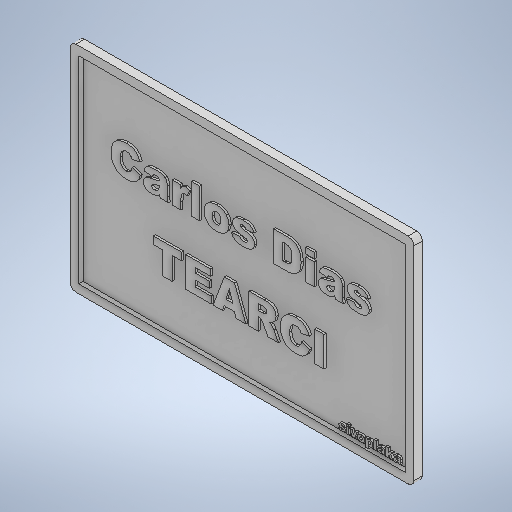
# Autodesk Inventor part: ID
Saved by Autodesk Inventor 2025.2 (Build 292293000, 293)
## iProperties
Created: 2025-01-22
Part Number: ID
Material: Generic
Document SubType Name: Modeling
Designer: Tony Dias
Density: 1 g/cm^3
Appearance: Default
Author: Tony Dias
## iProperties of the stored document ID_3DPrint.ipt
Created: 2025-01-22
Part Number: ID_3DPrint
Material: Generic
Document SubType Name: Modeling
Designer: Tony Dias
Density: 1 g/cm^3
Appearance: Default
Author: Tony Dias
Autodesk Inventor part; units mm, degrees
ref_plane "YZ Plane" through (0, 0, 0) normal (1, 0, 0) x (0, 1, 0)
ref_plane "XZ Plane" through (0, 0, 0) normal (0, 1, 0) x (-1, 0, 0)
ref_plane "XY Plane" through (0, 0, 0) normal (0, 0, 1) x (1, 0, 0)
sketch "Sketch1" plane through (0, 0, 0) normal (0, 0, 1) x (1, 0, 0)
  line L0 (-4, 2.5) -> (4, 2.5)
  line L1 (4, 2.5) -> (4, -2.5)
  line L2 (4, -2.5) -> (-4, -2.5)
  line L3 (-4, -2.5) -> (-4, 2.5)
  line L4 (-4, 2.5) -> (4, -2.5) construction
  line L5 (4, 2.5) -> (-4, -2.5) construction
  line L6 (-3.75, 2.3438) -> (3.75, -2.3438) construction
  line L7 (3.75, 2.3438) -> (-3.75, -2.3438) construction
  line L8 (3.8, -2.3) -> (-3.8, -2.3)
  line L9 (-3.8, 2.3) -> (-3.8, -2.3)
  line L10 (-3.8, 2.3) -> (3.8, 2.3)
  line L11 (3.8, 2.3) -> (3.8, -2.3)
  point P0 (0, 0)
  dimension "d0" = 8
  dimension "d1" = 5
  dimension "d2" = 7.5
  constraints: 24 end point, 4 midpoint, 3 horizontal, 3 perpendicular, 2 parallel, 1 point on line
  measures "d0" distance of L1.end L2.end
  measures "d1" distance of L0.end L1.end
  measures "d2" distance of L6.end L7.end
extrude "Extrusion1" add sketch "Sketch1" along normal blind 0.1 contours L8 L9 L10 L11
extrude "Extrusion2" add sketch "Sketch1" along normal blind 0.2
sketch "Sketch2" plane through (0, 0, 0) normal (0, 0, -1) x (-1, 0, 0)
  line L0 (-4, -2.5) -> (-4, 2.5) projected
  line L1 (-0.95, 0.4603) -> (-0.95, -0.4603) construction
  line L2 (-1.2, 0.4603) -> (-1.2, -0.4603)
  line L3 (-0.7, -0.4603) -> (-0.7, 0.4603)
  arc A0 (-0.7, 0.4603) -> (-1.2, 0.4603) centre (-0.95, 0.4603) ccw
  arc A1 (-1.2, -0.4603) -> (-0.7, -0.4603) centre (-0.95, -0.4603) ccw
  line L4 (0.95, 0.4603) -> (0.95, -0.4603) construction
  line L5 (0.7, 0.4603) -> (0.7, -0.4603)
  line L6 (1.2, -0.4603) -> (1.2, 0.4603)
  arc A2 (1.2, 0.4603) -> (0.7, 0.4603) centre (0.95, 0.4603) ccw
  arc A3 (0.7, -0.4603) -> (1.2, -0.4603) centre (0.95, -0.4603) ccw
  point P0 (0, 0)
  dimension "d13" = 0.5
  dimension "d15" = 0.5
  constraints: 16 end point, 8 point on circle, 8 tangent, 4 centre point, 2 parallel, 1 vertical
  measures "d13" diameter of A1
  measures "d15" diameter of A3
extrude "Extrusion3" add sketch "Sketch2" along normal blind 0.5
sketch "Sketch3" plane through (-1.2, -0.4603, 0) normal (-1, 0, 0) x (0, 0, 1)
  point P0 (0, 0.4603)
  point P1 (-0.2541, 0.4313)
hole "Hole1" at (-1.2, -0.029, -0.2541) direction (1, 0, 0) diameter 0.2 end through all
fillet "Face Fillet1" radius 0.133 1 edges at (0.95, 0.7103, -0.5)
fillet "Face Fillet2" radius 0.133 1 edges at (-0.95, 0.7103, -0.5)
sketch "Sketch4" plane through (0, 0, 0.2) normal (0, 0, 1) x (1, 0, 0)
  line L0 (-3.8117, 2.3101) -> (3.8117, 2.3101) construction
  line L1 (3.8117, 2.3101) -> (3.8117, -2.2966) construction
  line L2 (3.8117, -2.2966) -> (-3.8117, -2.2966) construction
  line L3 (-3.8117, -2.2966) -> (-3.8117, 2.3101) construction
  line L4 (2.2708, -1.8777) -> (3.7723, -1.8777) construction
  line L5 (3.7723, -1.8777) -> (3.7723, -2.2813) construction
  line L6 (3.7723, -2.2813) -> (2.2708, -2.2813) construction
  line L7 (2.2708, -2.2813) -> (2.2708, -1.8777) construction
  line L8 (-2.5069, 0.7143) -> (-2.3176, 0.657)
  spline S0 degree 2 poles (-2.3176, 0.657) (-2.3365, 0.5775) (-2.4187, 0.4704) (-2.5406, 0.4159) (-2.6343, 0.4159) knots 0 0 0 1 2 3 3 3
  spline S1 degree 2 poles (-2.6343, 0.4159) (-2.7488, 0.4159) (-2.893, 0.4826) (-2.9981, 0.6496) (-2.9981, 0.7797) knots 0 0 0 1 2 3 3 3
  spline S2 degree 2 poles (-2.9981, 0.7797) (-2.9981, 0.9535) (-2.8135, 1.1401) (-2.6444, 1.1401) knots 0 0 0 1 2 2 2
  spline S3 degree 2 poles (-2.6444, 1.1401) (-2.5123, 1.1401) (-2.3614, 1.033) (-2.3244, 0.9225) knots 0 0 0 1 2 2 2
  line L9 (-2.3244, 0.9225) -> (-2.5157, 0.8801)
  spline S4 degree 2 poles (-2.5157, 0.8801) (-2.5258, 0.9117) (-2.5366, 0.9265) knots 0 0 0 1 1 1
  spline S5 degree 2 poles (-2.5366, 0.9265) (-2.5548, 0.9515) (-2.6073, 0.9784) (-2.6397, 0.9784) knots 0 0 0 1 2 2 2
  spline S6 degree 2 poles (-2.6397, 0.9784) (-2.7124, 0.9784) (-2.7515, 0.9191) knots 0 0 0 1 1 1
  spline S7 degree 2 poles (-2.7515, 0.9191) (-2.7811, 0.8753) (-2.7811, 0.781) knots 0 0 0 1 1 1
  spline S8 degree 2 poles (-2.7811, 0.781) (-2.7811, 0.6645) (-2.7104, 0.5782) (-2.6464, 0.5782) knots 0 0 0 1 2 2 2
  spline S9 degree 2 poles (-2.6464, 0.5782) (-2.5844, 0.5782) (-2.5211, 0.6476) (-2.5069, 0.7143) knots 0 0 0 1 2 2 2
  line L10 (-2.0468, 0.7702) -> (-2.2327, 0.7898)
  spline S10 degree 2 poles (-2.2327, 0.7898) (-2.2219, 0.839) (-2.1829, 0.8949) (-2.1451, 0.9158) knots 0 0 0 1 2 2 2
  spline S11 degree 2 poles (-2.1451, 0.9158) (-2.1189, 0.9306) (-2.0252, 0.9468) (-1.9706, 0.9468) knots 0 0 0 1 2 2 2
  spline S12 degree 2 poles (-1.9706, 0.9468) (-1.8837, 0.9468) (-1.778, 0.9272) (-1.7423, 0.8962) knots 0 0 0 1 2 2 2
  spline S13 degree 2 poles (-1.7423, 0.8962) (-1.7173, 0.8747) (-1.689, 0.7958) (-1.689, 0.7601) knots 0 0 0 1 2 2 2
  line L11 (-1.689, 0.7601) -> (-1.689, 0.5358)
  spline S14 degree 2 poles (-1.689, 0.5358) (-1.689, 0.5001) (-1.6803, 0.4596) (-1.6648, 0.428) knots 0 0 0 1 2 2 2
  line L12 (-1.6648, 0.428) -> (-1.8474, 0.428)
  spline S15 degree 2 poles (-1.8474, 0.428) (-1.8581, 0.4475) (-1.8649, 0.4677) (-1.8682, 0.49) knots 0 0 0 1 2 2 2
  spline S16 degree 2 poles (-1.8682, 0.49) (-1.906, 0.4536) (-1.9437, 0.4374) knots 0 0 0 1 1 1
  spline S17 degree 2 poles (-1.9437, 0.4374) (-1.9956, 0.4165) (-2.0636, 0.4165) knots 0 0 0 1 1 1
  spline S18 degree 2 poles (-2.0636, 0.4165) (-2.1546, 0.4165) (-2.2482, 0.5007) (-2.2482, 0.5621) knots 0 0 0 1 2 2 2
  spline S19 degree 2 poles (-2.2482, 0.5621) (-2.2482, 0.62) (-2.2145, 0.657) knots 0 0 0 1 1 1
  spline S20 degree 2 poles (-2.2145, 0.657) (-2.1802, 0.6941) (-2.0892, 0.7123) knots 0 0 0 1 1 1
  spline S21 degree 2 poles (-2.0892, 0.7123) (-1.9801, 0.7345) (-1.9154, 0.752) (-1.879, 0.7662) knots 0 0 0 1 2 2 2
  spline S22 degree 2 poles (-1.879, 0.7662) (-1.879, 0.8019) (-1.9087, 0.8309) (-1.9457, 0.8309) knots 0 0 0 1 2 2 2
  spline S23 degree 2 poles (-1.9457, 0.8309) (-1.9929, 0.8309) (-2.0171, 0.8154) knots 0 0 0 1 1 1
  spline S24 degree 2 poles (-2.0171, 0.8154) (-2.0353, 0.8032) (-2.0468, 0.7702) knots 0 0 0 1 1 1
  spline S25 degree 2 poles (-1.879, 0.6685) (-1.9188, 0.6544) (-1.9626, 0.6429) knots 0 0 0 1 1 1
  spline S26 degree 2 poles (-1.9626, 0.6429) (-2.0218, 0.6274) (-2.0373, 0.6119) knots 0 0 0 1 1 1
  spline S27 degree 2 poles (-2.0373, 0.6119) (-2.0535, 0.5964) (-2.0535, 0.5762) knots 0 0 0 1 1 1
  spline S28 degree 2 poles (-2.0535, 0.5762) (-2.0535, 0.5533) (-2.0218, 0.5243) (-1.9909, 0.5243) knots 0 0 0 1 2 2 2
  spline S29 degree 2 poles (-1.9909, 0.5243) (-1.9578, 0.5243) (-1.9026, 0.556) (-1.879, 0.6011) (-1.879, 0.6375) knots 0 0 0 1 2 3 3 3
  line L13 (-1.879, 0.6375) -> (-1.879, 0.6685)
  line L14 (-1.5698, 0.9353) -> (-1.3879, 0.9353)
  line L15 (-1.3879, 0.9353) -> (-1.3879, 0.8524)
  spline S30 degree 2 poles (-1.3879, 0.8524) (-1.3616, 0.9063) (-1.3057, 0.9468) (-1.2646, 0.9468) knots 0 0 0 1 2 2 2
  spline S31 degree 2 poles (-1.2646, 0.9468) (-1.2215, 0.9468) (-1.1703, 0.9198) knots 0 0 0 1 1 1
  line L16 (-1.1703, 0.9198) -> (-1.2302, 0.7817)
  spline S32 degree 2 poles (-1.2302, 0.7817) (-1.2646, 0.7958) (-1.2848, 0.7958) knots 0 0 0 1 1 1
  spline S33 degree 2 poles (-1.2848, 0.7958) (-1.3232, 0.7958) (-1.3441, 0.7642) knots 0 0 0 1 1 1
  spline S34 degree 2 poles (-1.3441, 0.7642) (-1.3744, 0.7197) (-1.3744, 0.5978) knots 0 0 0 1 1 1
  line L17 (-1.3744, 0.5978) -> (-1.3744, 0.428)
  line L18 (-1.3744, 0.428) -> (-1.5698, 0.428)
  line L19 (-1.5698, 0.428) -> (-1.5698, 0.9353)
  line L20 (-1.1305, 1.128) -> (-0.9358, 1.128)
  line L21 (-0.9358, 1.128) -> (-0.9358, 0.428)
  line L22 (-0.9358, 0.428) -> (-1.1305, 0.428)
  line L23 (-1.1305, 0.428) -> (-1.1305, 1.128)
  spline S35 degree 2 poles (-0.8347, 0.68) (-0.8347, 0.7965) (-0.6784, 0.9468) (-0.545, 0.9468) knots 0 0 0 1 2 2 2
  spline S36 degree 2 poles (-0.545, 0.9468) (-0.3928, 0.9468) (-0.3153, 0.8585) knots 0 0 0 1 1 1
  spline S37 degree 2 poles (-0.3153, 0.8585) (-0.2526, 0.7871) (-0.2526, 0.6833) knots 0 0 0 1 1 1
  spline S38 degree 2 poles (-0.2526, 0.6833) (-0.2526, 0.5661) (-0.4076, 0.4165) (-0.5444, 0.4165) knots 0 0 0 1 2 2 2
  spline S39 degree 2 poles (-0.5444, 0.4165) (-0.667, 0.4165) (-0.7424, 0.4785) knots 0 0 0 1 1 1
  spline S40 degree 2 poles (-0.7424, 0.4785) (-0.8347, 0.5553) (-0.8347, 0.68) knots 0 0 0 1 1 1
  spline S41 degree 2 poles (-0.64, 0.6806) (-0.64, 0.6126) (-0.5855, 0.5479) (-0.5437, 0.5479) knots 0 0 0 1 2 2 2
  spline S42 degree 2 poles (-0.5437, 0.5479) (-0.5019, 0.5479) (-0.448, 0.6119) (-0.448, 0.6827) knots 0 0 0 1 2 2 2
  spline S43 degree 2 poles (-0.448, 0.6827) (-0.448, 0.748) (-0.5026, 0.8127) (-0.5423, 0.8127) knots 0 0 0 1 2 2 2
  spline S44 degree 2 poles (-0.5423, 0.8127) (-0.5848, 0.8127) (-0.64, 0.7473) (-0.64, 0.6806) knots 0 0 0 1 2 2 2
  line L24 (-0.1927, 0.5688) -> (0, 0.587)
  spline S45 degree 2 poles (0, 0.587) (0.0121, 0.5526) (0.0552, 0.523) (0.091, 0.523) knots 0 0 0 1 2 2 2
  spline S46 degree 2 poles (0.091, 0.523) (0.1307, 0.523) (0.1523, 0.5398) knots 0 0 0 1 1 1
  spline S47 degree 2 poles (0.1523, 0.5398) (0.1691, 0.5519) (0.1691, 0.5708) knots 0 0 0 1 1 1
  spline S48 degree 2 poles (0.1691, 0.5708) (0.1691, 0.5917) (0.1469, 0.6032) knots 0 0 0 1 1 1
  spline S49 degree 2 poles (0.1469, 0.6032) (0.1307, 0.6112) (0.0633, 0.6234) knots 0 0 0 1 1 1
  spline S50 degree 2 poles (0.0633, 0.6234) (-0.0384, 0.6409) (-0.1172, 0.6712) (-0.1711, 0.7426) (-0.1711, 0.7884) knots 0 0 0 1 2 3 3 3
  spline S51 degree 2 poles (-0.1711, 0.7884) (-0.1711, 0.8383) (-0.1125, 0.911) (-0.0108, 0.9468) (0.0755, 0.9468) knots 0 0 0 1 2 3 3 3
  spline S52 degree 2 poles (0.0755, 0.9468) (0.1664, 0.9468) (0.2526, 0.9191) (0.3106, 0.8612) (0.3295, 0.8113) knots 0 0 0 1 2 3 3 3
  line L25 (0.3295, 0.8113) -> (0.1449, 0.7931)
  spline S53 degree 2 poles (0.1449, 0.7931) (0.1374, 0.8174) (0.1213, 0.8288) knots 0 0 0 1 1 1
  spline S54 degree 2 poles (0.1213, 0.8288) (0.0984, 0.8443) (0.0654, 0.8443) knots 0 0 0 1 1 1
  spline S55 degree 2 poles (0.0654, 0.8443) (0.033, 0.8443) (0.0027, 0.8208) (0.0027, 0.8039) knots 0 0 0 1 2 2 2
  spline S56 degree 2 poles (0.0027, 0.8039) (0.0027, 0.7857) (0.0222, 0.7763) knots 0 0 0 1 1 1
  spline S57 degree 2 poles (0.0222, 0.7763) (0.0411, 0.7662) (0.1051, 0.7588) knots 0 0 0 1 1 1
  spline S58 degree 2 poles (0.1051, 0.7588) (0.2021, 0.748) (0.2971, 0.7089) (0.347, 0.6362) (0.347, 0.593) knots 0 0 0 1 2 3 3 3
  spline S59 degree 2 poles (0.347, 0.593) (0.347, 0.5486) (0.2937, 0.4657) (0.1799, 0.4165) (0.0815, 0.4165) knots 0 0 0 1 2 3 3 3
  spline S60 degree 2 poles (0.0815, 0.4165) (-0.0579, 0.4165) (-0.1758, 0.496) (-0.1927, 0.5688) knots 0 0 0 1 2 2 2
  line L26 (0.7815, 1.128) -> (1.1029, 1.128)
  spline S61 degree 2 poles (1.1029, 1.128) (1.1979, 1.128) (1.3151, 1.0761) (1.3912, 0.9798) (1.4256, 0.8518) (1.4256, 0.7803) knots 0 0 0 1 2 3 4 4 4
  spline S62 degree 2 poles (1.4256, 0.7803) (1.4256, 0.6678) (1.3744, 0.5445) (1.2841, 0.461) (1.2316, 0.4468) knots 0 0 0 1 2 3 3 3
  spline S63 degree 2 poles (1.2316, 0.4468) (1.1608, 0.428) (1.1029, 0.428) knots 0 0 0 1 1 1
  line L27 (1.1029, 0.428) -> (0.7815, 0.428)
  line L28 (0.7815, 0.428) -> (0.7815, 1.128)
  line L29 (0.9978, 0.9697) -> (0.9978, 0.587)
  line L30 (0.9978, 0.587) -> (1.051, 0.587)
  spline S64 degree 2 poles (1.051, 0.587) (1.1184, 0.587) (1.1756, 0.6173) (1.208, 0.6921) (1.208, 0.7763) knots 0 0 0 1 2 3 3 3
  spline S65 degree 2 poles (1.208, 0.7763) (1.208, 0.8875) (1.1352, 0.9697) (1.0517, 0.9697) knots 0 0 0 1 2 2 2
  line L31 (1.0517, 0.9697) -> (0.9978, 0.9697)
  line L32 (1.5341, 0.9353) -> (1.7288, 0.9353)
  line L33 (1.7288, 0.9353) -> (1.7288, 0.428)
  line L34 (1.7288, 0.428) -> (1.5341, 0.428)
  line L35 (1.5341, 0.428) -> (1.5341, 0.9353)
  line L36 (1.5341, 1.128) -> (1.7288, 1.128)
  line L37 (1.7288, 1.128) -> (1.7288, 0.9959)
  line L38 (1.7288, 0.9959) -> (1.5341, 0.9959)
  line L39 (1.5341, 0.9959) -> (1.5341, 1.128)
  line L40 (2.0306, 0.7702) -> (1.8447, 0.7898)
  spline S66 degree 2 poles (1.8447, 0.7898) (1.8554, 0.839) (1.8945, 0.8949) (1.9322, 0.9158) knots 0 0 0 1 2 2 2
  spline S67 degree 2 poles (1.9322, 0.9158) (1.9585, 0.9306) (2.0522, 0.9468) (2.1067, 0.9468) knots 0 0 0 1 2 2 2
  spline S68 degree 2 poles (2.1067, 0.9468) (2.1936, 0.9468) (2.2994, 0.9272) (2.3351, 0.8962) knots 0 0 0 1 2 2 2
  spline S69 degree 2 poles (2.3351, 0.8962) (2.3601, 0.8747) (2.3884, 0.7958) (2.3884, 0.7601) knots 0 0 0 1 2 2 2
  line L41 (2.3884, 0.7601) -> (2.3884, 0.5358)
  spline S70 degree 2 poles (2.3884, 0.5358) (2.3884, 0.5001) (2.3971, 0.4596) (2.4126, 0.428) knots 0 0 0 1 2 2 2
  line L42 (2.4126, 0.428) -> (2.23, 0.428)
  spline S71 degree 2 poles (2.23, 0.428) (2.2192, 0.4475) (2.2125, 0.4677) (2.2091, 0.49) knots 0 0 0 1 2 2 2
  spline S72 degree 2 poles (2.2091, 0.49) (2.1714, 0.4536) (2.1337, 0.4374) knots 0 0 0 1 1 1
  spline S73 degree 2 poles (2.1337, 0.4374) (2.0818, 0.4165) (2.0138, 0.4165) knots 0 0 0 1 1 1
  spline S74 degree 2 poles (2.0138, 0.4165) (1.9228, 0.4165) (1.8292, 0.5007) (1.8292, 0.5621) knots 0 0 0 1 2 2 2
  spline S75 degree 2 poles (1.8292, 0.5621) (1.8292, 0.62) (1.8628, 0.657) knots 0 0 0 1 1 1
  spline S76 degree 2 poles (1.8628, 0.657) (1.8972, 0.6941) (1.9882, 0.7123) knots 0 0 0 1 1 1
  spline S77 degree 2 poles (1.9882, 0.7123) (2.0973, 0.7345) (2.162, 0.752) (2.1984, 0.7662) knots 0 0 0 1 2 2 2
  spline S78 degree 2 poles (2.1984, 0.7662) (2.1984, 0.8019) (2.1687, 0.8309) (2.1317, 0.8309) knots 0 0 0 1 2 2 2
  spline S79 degree 2 poles (2.1317, 0.8309) (2.0845, 0.8309) (2.0603, 0.8154) knots 0 0 0 1 1 1
  spline S80 degree 2 poles (2.0603, 0.8154) (2.0421, 0.8032) (2.0306, 0.7702) knots 0 0 0 1 1 1
  spline S81 degree 2 poles (2.1984, 0.6685) (2.1586, 0.6544) (2.1148, 0.6429) knots 0 0 0 1 1 1
  spline S82 degree 2 poles (2.1148, 0.6429) (2.0555, 0.6274) (2.04, 0.6119) knots 0 0 0 1 1 1
  spline S83 degree 2 poles (2.04, 0.6119) (2.0239, 0.5964) (2.0239, 0.5762) knots 0 0 0 1 1 1
  spline S84 degree 2 poles (2.0239, 0.5762) (2.0239, 0.5533) (2.0555, 0.5243) (2.0865, 0.5243) knots 0 0 0 1 2 2 2
  spline S85 degree 2 poles (2.0865, 0.5243) (2.1195, 0.5243) (2.1748, 0.556) (2.1984, 0.6011) (2.1984, 0.6375) knots 0 0 0 1 2 3 3 3
  line L43 (2.1984, 0.6375) -> (2.1984, 0.6685)
  line L44 (2.4712, 0.5688) -> (2.6639, 0.587)
  spline S86 degree 2 poles (2.6639, 0.587) (2.676, 0.5526) (2.7192, 0.523) (2.7549, 0.523) knots 0 0 0 1 2 2 2
  spline S87 degree 2 poles (2.7549, 0.523) (2.7946, 0.523) (2.8162, 0.5398) knots 0 0 0 1 1 1
  spline S88 degree 2 poles (2.8162, 0.5398) (2.833, 0.5519) (2.833, 0.5708) knots 0 0 0 1 1 1
  spline S89 degree 2 poles (2.833, 0.5708) (2.833, 0.5917) (2.8108, 0.6032) knots 0 0 0 1 1 1
  spline S90 degree 2 poles (2.8108, 0.6032) (2.7946, 0.6112) (2.7272, 0.6234) knots 0 0 0 1 1 1
  spline S91 degree 2 poles (2.7272, 0.6234) (2.6255, 0.6409) (2.5467, 0.6712) (2.4928, 0.7426) (2.4928, 0.7884) knots 0 0 0 1 2 3 3 3
  spline S92 degree 2 poles (2.4928, 0.7884) (2.4928, 0.8383) (2.5514, 0.911) (2.6531, 0.9468) (2.7394, 0.9468) knots 0 0 0 1 2 3 3 3
  spline S93 degree 2 poles (2.7394, 0.9468) (2.8303, 0.9468) (2.9166, 0.9191) (2.9745, 0.8612) (2.9934, 0.8113) knots 0 0 0 1 2 3 3 3
  line L45 (2.9934, 0.8113) -> (2.8088, 0.7931)
  spline S94 degree 2 poles (2.8088, 0.7931) (2.8013, 0.8174) (2.7852, 0.8288) knots 0 0 0 1 1 1
  spline S95 degree 2 poles (2.7852, 0.8288) (2.7623, 0.8443) (2.7293, 0.8443) knots 0 0 0 1 1 1
  spline S96 degree 2 poles (2.7293, 0.8443) (2.6969, 0.8443) (2.6666, 0.8208) (2.6666, 0.8039) knots 0 0 0 1 2 2 2
  spline S97 degree 2 poles (2.6666, 0.8039) (2.6666, 0.7857) (2.6861, 0.7763) knots 0 0 0 1 1 1
  spline S98 degree 2 poles (2.6861, 0.7763) (2.705, 0.7662) (2.769, 0.7588) knots 0 0 0 1 1 1
  spline S99 degree 2 poles (2.769, 0.7588) (2.866, 0.748) (2.961, 0.7089) (3.0109, 0.6362) (3.0109, 0.593) knots 0 0 0 1 2 3 3 3
  spline S100 degree 2 poles (3.0109, 0.593) (3.0109, 0.5486) (2.9577, 0.4657) (2.8438, 0.4165) (2.7454, 0.4165) knots 0 0 0 1 2 3 3 3
  spline S101 degree 2 poles (2.7454, 0.4165) (2.606, 0.4165) (2.4881, 0.496) (2.4712, 0.5688) knots 0 0 0 1 2 2 2
  line L46 (-2.0168, -0.4144) -> (-1.3586, -0.4144)
  line L47 (-1.3586, -0.4144) -> (-1.3586, -0.5875)
  line L48 (-1.3586, -0.5875) -> (-1.5795, -0.5875)
  line L49 (-1.5795, -0.5875) -> (-1.5795, -1.1144)
  line L50 (-1.5795, -1.1144) -> (-1.7958, -1.1144)
  line L51 (-1.7958, -1.1144) -> (-1.7958, -0.5875)
  line L52 (-1.7958, -0.5875) -> (-2.0168, -0.5875)
  line L53 (-2.0168, -0.5875) -> (-2.0168, -0.4144)
  line L54 (-1.2609, -0.4144) -> (-0.6815, -0.4144)
  line L55 (-0.6815, -0.4144) -> (-0.6815, -0.564)
  line L56 (-0.6815, -0.564) -> (-1.0439, -0.564)
  line L57 (-1.0439, -0.564) -> (-1.0439, -0.6751)
  line L58 (-1.0439, -0.6751) -> (-0.7077, -0.6751)
  line L59 (-0.7077, -0.6751) -> (-0.7077, -0.818)
  line L60 (-0.7077, -0.818) -> (-1.0439, -0.818)
  line L61 (-1.0439, -0.818) -> (-1.0439, -0.9561)
  line L62 (-1.0439, -0.9561) -> (-0.6707, -0.9561)
  line L63 (-0.6707, -0.9561) -> (-0.6707, -1.1144)
  line L64 (-0.6707, -1.1144) -> (-1.2609, -1.1144)
  line L65 (-1.2609, -1.1144) -> (-1.2609, -0.4144)
  line L66 (-0.1236, -0.9985) -> (-0.3695, -0.9985)
  line L67 (-0.3695, -0.9985) -> (-0.4039, -1.1144)
  line L68 (-0.4039, -1.1144) -> (-0.6249, -1.1144)
  line L69 (-0.6249, -1.1144) -> (-0.3615, -0.4144)
  line L70 (-0.3615, -0.4144) -> (-0.125, -0.4144)
  line L71 (-0.125, -0.4144) -> (0.1378, -1.1144)
  line L72 (0.1378, -1.1144) -> (-0.0886, -1.1144)
  line L73 (-0.0886, -1.1144) -> (-0.1236, -0.9985)
  line L74 (-0.1688, -0.8469) -> (-0.2456, -0.5956)
  line L75 (-0.2456, -0.5956) -> (-0.3224, -0.8469)
  line L76 (-0.3224, -0.8469) -> (-0.1688, -0.8469)
  line L77 (0.2105, -1.1144) -> (0.2105, -0.4144)
  line L78 (0.2105, -0.4144) -> (0.571, -0.4144)
  spline S102 degree 2 poles (0.571, -0.4144) (0.6707, -0.4144) (0.7771, -0.4488) (0.8418, -0.5417) (0.8418, -0.6084) knots 0 0 0 1 2 3 3 3
  spline S103 degree 2 poles (0.8418, -0.6084) (0.8418, -0.667) (0.792, -0.7513) (0.7488, -0.7775) knots 0 0 0 1 2 2 2
  spline S104 degree 2 poles (0.7488, -0.7775) (0.7212, -0.7944) (0.6727, -0.8052) knots 0 0 0 1 1 1
  spline S105 degree 2 poles (0.6727, -0.8052) (0.7111, -0.818) (0.7293, -0.8308) knots 0 0 0 1 1 1
  spline S106 degree 2 poles (0.7293, -0.8308) (0.7408, -0.8395) (0.7859, -0.8961) (0.794, -0.9116) knots 0 0 0 1 2 2 2
  line L79 (0.794, -0.9116) -> (0.8984, -1.1144)
  line L80 (0.8984, -1.1144) -> (0.6538, -1.1144)
  line L81 (0.6538, -1.1144) -> (0.5386, -0.9001)
  spline S107 degree 2 poles (0.5386, -0.9001) (0.5171, -0.8591) (0.5002, -0.8463) knots 0 0 0 1 1 1
  spline S108 degree 2 poles (0.5002, -0.8463) (0.4767, -0.8301) (0.447, -0.8301) knots 0 0 0 1 1 1
  line L82 (0.447, -0.8301) -> (0.4282, -0.8301)
  line L83 (0.4282, -0.8301) -> (0.4282, -1.1144)
  line L84 (0.4282, -1.1144) -> (0.2105, -1.1144)
  line L85 (0.4282, -0.698) -> (0.5191, -0.698)
  spline S109 degree 2 poles (0.5191, -0.698) (0.5333, -0.698) (0.5757, -0.6886) knots 0 0 0 1 1 1
  spline S110 degree 2 poles (0.5757, -0.6886) (0.5973, -0.6839) (0.6242, -0.6488) (0.6242, -0.6259) knots 0 0 0 1 2 2 2
  spline S111 degree 2 poles (0.6242, -0.6259) (0.6242, -0.5923) (0.5818, -0.5559) (0.5225, -0.5559) knots 0 0 0 1 2 2 2
  line L86 (0.5225, -0.5559) -> (0.4282, -0.5559)
  line L87 (0.4282, -0.5559) -> (0.4282, -0.698)
  line L88 (1.4347, -0.8281) -> (1.624, -0.8853)
  spline S112 degree 2 poles (1.624, -0.8853) (1.6051, -0.9648) (1.523, -1.0719) (1.401, -1.1265) (1.3074, -1.1265) knots 0 0 0 1 2 3 3 3
  spline S113 degree 2 poles (1.3074, -1.1265) (1.1928, -1.1265) (1.0487, -1.0598) (0.9436, -0.8927) (0.9436, -0.7627) knots 0 0 0 1 2 3 3 3
  spline S114 degree 2 poles (0.9436, -0.7627) (0.9436, -0.5889) (1.1282, -0.4023) (1.2973, -0.4023) knots 0 0 0 1 2 2 2
  spline S115 degree 2 poles (1.2973, -0.4023) (1.4293, -0.4023) (1.5802, -0.5094) (1.6173, -0.6199) knots 0 0 0 1 2 2 2
  line L89 (1.6173, -0.6199) -> (1.4259, -0.6623)
  spline S116 degree 2 poles (1.4259, -0.6623) (1.4158, -0.6307) (1.4051, -0.6158) knots 0 0 0 1 1 1
  spline S117 degree 2 poles (1.4051, -0.6158) (1.3869, -0.5909) (1.3343, -0.564) (1.302, -0.564) knots 0 0 0 1 2 2 2
  spline S118 degree 2 poles (1.302, -0.564) (1.2292, -0.564) (1.1901, -0.6232) knots 0 0 0 1 1 1
  spline S119 degree 2 poles (1.1901, -0.6232) (1.1605, -0.667) (1.1605, -0.7614) knots 0 0 0 1 1 1
  spline S120 degree 2 poles (1.1605, -0.7614) (1.1605, -0.8779) (1.2312, -0.9642) (1.2952, -0.9642) knots 0 0 0 1 2 2 2
  spline S121 degree 2 poles (1.2952, -0.9642) (1.3572, -0.9642) (1.4205, -0.8948) (1.4347, -0.8281) knots 0 0 0 1 2 2 2
  line L90 (1.7385, -0.4144) -> (1.9555, -0.4144)
  line L91 (1.9555, -0.4144) -> (1.9555, -1.1144)
  line L92 (1.9555, -1.1144) -> (1.7385, -1.1144)
  line L93 (1.7385, -1.1144) -> (1.7385, -0.4144)
  line L94 (2.2983, -2.1117) -> (2.3533, -2.1065)
  spline S122 degree 2 poles (2.3533, -2.1065) (2.3568, -2.1163) (2.3691, -2.1248) (2.3793, -2.1248) knots 0 0 0 1 2 2 2
  spline S123 degree 2 poles (2.3793, -2.1248) (2.3907, -2.1248) (2.3968, -2.12) knots 0 0 0 1 1 1
  spline S124 degree 2 poles (2.3968, -2.12) (2.4017, -2.1165) (2.4017, -2.1111) knots 0 0 0 1 1 1
  spline S125 degree 2 poles (2.4017, -2.1111) (2.4017, -2.1052) (2.3953, -2.1019) knots 0 0 0 1 1 1
  spline S126 degree 2 poles (2.3953, -2.1019) (2.3907, -2.0996) (2.3714, -2.0961) knots 0 0 0 1 1 1
  spline S127 degree 2 poles (2.3714, -2.0961) (2.3424, -2.0911) (2.3198, -2.0825) (2.3044, -2.0621) (2.3044, -2.049) knots 0 0 0 1 2 3 3 3
  spline S128 degree 2 poles (2.3044, -2.049) (2.3044, -2.0347) (2.3212, -2.0139) (2.3503, -2.0037) (2.3749, -2.0037) knots 0 0 0 1 2 3 3 3
  spline S129 degree 2 poles (2.3749, -2.0037) (2.4009, -2.0037) (2.4255, -2.0116) (2.4421, -2.0282) (2.4475, -2.0424) knots 0 0 0 1 2 3 3 3
  line L95 (2.4475, -2.0424) -> (2.3947, -2.0476)
  spline S130 degree 2 poles (2.3947, -2.0476) (2.3926, -2.0407) (2.388, -2.0374) knots 0 0 0 1 1 1
  spline S131 degree 2 poles (2.388, -2.0374) (2.3814, -2.033) (2.372, -2.033) knots 0 0 0 1 1 1
  spline S132 degree 2 poles (2.372, -2.033) (2.3628, -2.033) (2.3541, -2.0397) (2.3541, -2.0445) knots 0 0 0 1 2 2 2
  spline S133 degree 2 poles (2.3541, -2.0445) (2.3541, -2.0497) (2.3597, -2.0524) knots 0 0 0 1 1 1
  spline S134 degree 2 poles (2.3597, -2.0524) (2.3651, -2.0553) (2.3834, -2.0574) knots 0 0 0 1 1 1
  spline S135 degree 2 poles (2.3834, -2.0574) (2.4111, -2.0605) (2.4382, -2.0717) (2.4525, -2.0925) (2.4525, -2.1048) knots 0 0 0 1 2 3 3 3
  spline S136 degree 2 poles (2.4525, -2.1048) (2.4525, -2.1175) (2.4373, -2.1412) (2.4047, -2.1552) (2.3766, -2.1552) knots 0 0 0 1 2 3 3 3
  spline S137 degree 2 poles (2.3766, -2.1552) (2.3368, -2.1552) (2.3031, -2.1325) (2.2983, -2.1117) knots 0 0 0 1 2 2 2
  line L96 (2.481, -2.007) -> (2.5366, -2.007)
  line L97 (2.5366, -2.007) -> (2.5366, -2.152)
  line L98 (2.5366, -2.152) -> (2.481, -2.152)
  line L99 (2.481, -2.152) -> (2.481, -2.007)
  line L100 (2.481, -1.952) -> (2.5366, -1.952)
  line L101 (2.5366, -1.952) -> (2.5366, -1.9897)
  line L102 (2.5366, -1.9897) -> (2.481, -1.9897)
  line L103 (2.481, -1.9897) -> (2.481, -1.952)
  line L104 (2.5556, -2.007) -> (2.6134, -2.007)
  line L105 (2.6134, -2.007) -> (2.6417, -2.0988)
  line L106 (2.6417, -2.0988) -> (2.6708, -2.007)
  line L107 (2.6708, -2.007) -> (2.7268, -2.007)
  line L108 (2.7268, -2.007) -> (2.6652, -2.152)
  line L109 (2.6652, -2.152) -> (2.6159, -2.152)
  line L110 (2.6159, -2.152) -> (2.5556, -2.007)
  spline S138 degree 2 poles (2.736, -2.08) (2.736, -2.0467) (2.7807, -2.0037) (2.8188, -2.0037) knots 0 0 0 1 2 2 2
  spline S139 degree 2 poles (2.8188, -2.0037) (2.8623, -2.0037) (2.8844, -2.0289) knots 0 0 0 1 1 1
  spline S140 degree 2 poles (2.8844, -2.0289) (2.9023, -2.0494) (2.9023, -2.079) knots 0 0 0 1 1 1
  spline S141 degree 2 poles (2.9023, -2.079) (2.9023, -2.1125) (2.8581, -2.1552) (2.819, -2.1552) knots 0 0 0 1 2 2 2
  spline S142 degree 2 poles (2.819, -2.1552) (2.7839, -2.1552) (2.7624, -2.1375) knots 0 0 0 1 1 1
  spline S143 degree 2 poles (2.7624, -2.1375) (2.736, -2.1156) (2.736, -2.08) knots 0 0 0 1 1 1
  spline S144 degree 2 poles (2.7916, -2.0798) (2.7916, -2.0992) (2.8072, -2.1177) (2.8192, -2.1177) knots 0 0 0 1 2 2 2
  spline S145 degree 2 poles (2.8192, -2.1177) (2.8311, -2.1177) (2.8465, -2.0994) (2.8465, -2.0792) knots 0 0 0 1 2 2 2
  spline S146 degree 2 poles (2.8465, -2.0792) (2.8465, -2.0605) (2.8309, -2.042) (2.8196, -2.042) knots 0 0 0 1 2 2 2
  spline S147 degree 2 poles (2.8196, -2.042) (2.8074, -2.042) (2.7916, -2.0607) (2.7916, -2.0798) knots 0 0 0 1 2 2 2
  line L111 (2.9297, -2.207) -> (2.9297, -2.007)
  line L112 (2.9297, -2.007) -> (2.9816, -2.007)
  line L113 (2.9816, -2.007) -> (2.9816, -2.0284)
  spline S148 degree 2 poles (2.9816, -2.0284) (2.9924, -2.0149) (3.0013, -2.0101) knots 0 0 0 1 1 1
  spline S149 degree 2 poles (3.0013, -2.0101) (3.0136, -2.0037) (3.0282, -2.0037) knots 0 0 0 1 1 1
  spline S150 degree 2 poles (3.0282, -2.0037) (3.0573, -2.0037) (3.089, -2.0482) (3.089, -2.0809) knots 0 0 0 1 2 2 2
  spline S151 degree 2 poles (3.089, -2.0809) (3.089, -2.1171) (3.0544, -2.1552) (3.028, -2.1552) knots 0 0 0 1 2 2 2
  spline S152 degree 2 poles (3.028, -2.1552) (3.0151, -2.1552) (2.994, -2.1466) (2.9857, -2.1379) knots 0 0 0 1 2 2 2
  line L114 (2.9857, -2.1379) -> (2.9857, -2.207)
  line L115 (2.9857, -2.207) -> (2.9297, -2.207)
  spline S153 degree 2 poles (2.9853, -2.0798) (2.9853, -2.0971) (2.9997, -2.1136) (3.0107, -2.1136) knots 0 0 0 1 2 2 2
  spline S154 degree 2 poles (3.0107, -2.1136) (3.0203, -2.1136) (3.0334, -2.0977) (3.0334, -2.0786) knots 0 0 0 1 2 2 2
  spline S155 degree 2 poles (3.0334, -2.0786) (3.0334, -2.0611) (3.0197, -2.0445) (3.0099, -2.0445) knots 0 0 0 1 2 2 2
  spline S156 degree 2 poles (3.0099, -2.0445) (2.9993, -2.0445) (2.9853, -2.0611) (2.9853, -2.0798) knots 0 0 0 1 2 2 2
  line L116 (3.1177, -1.952) -> (3.1734, -1.952)
  line L117 (3.1734, -1.952) -> (3.1734, -2.152)
  line L118 (3.1734, -2.152) -> (3.1177, -2.152)
  line L119 (3.1177, -2.152) -> (3.1177, -1.952)
  line L120 (3.2598, -2.0542) -> (3.2067, -2.0486)
  spline S157 degree 2 poles (3.2067, -2.0486) (3.2097, -2.0345) (3.2209, -2.0186) (3.2317, -2.0126) knots 0 0 0 1 2 2 2
  spline S158 degree 2 poles (3.2317, -2.0126) (3.2392, -2.0084) (3.2659, -2.0037) (3.2815, -2.0037) knots 0 0 0 1 2 2 2
  spline S159 degree 2 poles (3.2815, -2.0037) (3.3064, -2.0037) (3.3366, -2.0093) (3.3468, -2.0182) knots 0 0 0 1 2 2 2
  spline S160 degree 2 poles (3.3468, -2.0182) (3.3539, -2.0243) (3.362, -2.0469) (3.362, -2.0571) knots 0 0 0 1 2 2 2
  line L121 (3.362, -2.0571) -> (3.362, -2.1212)
  spline S161 degree 2 poles (3.362, -2.1212) (3.362, -2.1314) (3.3645, -2.1429) (3.3689, -2.152) knots 0 0 0 1 2 2 2
  line L122 (3.3689, -2.152) -> (3.3168, -2.152)
  spline S162 degree 2 poles (3.3168, -2.152) (3.3137, -2.1464) (3.3118, -2.1406) (3.3108, -2.1342) knots 0 0 0 1 2 2 2
  spline S163 degree 2 poles (3.3108, -2.1342) (3.3, -2.1446) (3.2892, -2.1493) knots 0 0 0 1 1 1
  spline S164 degree 2 poles (3.2892, -2.1493) (3.2744, -2.1552) (3.255, -2.1552) knots 0 0 0 1 1 1
  spline S165 degree 2 poles (3.255, -2.1552) (3.229, -2.1552) (3.2022, -2.1312) (3.2022, -2.1136) knots 0 0 0 1 2 2 2
  spline S166 degree 2 poles (3.2022, -2.1136) (3.2022, -2.0971) (3.2119, -2.0865) knots 0 0 0 1 1 1
  spline S167 degree 2 poles (3.2119, -2.0865) (3.2217, -2.0759) (3.2477, -2.0707) knots 0 0 0 1 1 1
  spline S168 degree 2 poles (3.2477, -2.0707) (3.2788, -2.0644) (3.2973, -2.0594) (3.3077, -2.0553) knots 0 0 0 1 2 2 2
  spline S169 degree 2 poles (3.3077, -2.0553) (3.3077, -2.0451) (3.2992, -2.0368) (3.2887, -2.0368) knots 0 0 0 1 2 2 2
  spline S170 degree 2 poles (3.2887, -2.0368) (3.2752, -2.0368) (3.2683, -2.0413) knots 0 0 0 1 1 1
  spline S171 degree 2 poles (3.2683, -2.0413) (3.2631, -2.0447) (3.2598, -2.0542) knots 0 0 0 1 1 1
  spline S172 degree 2 poles (3.3077, -2.0832) (3.2964, -2.0873) (3.2838, -2.0905) knots 0 0 0 1 1 1
  spline S173 degree 2 poles (3.2838, -2.0905) (3.2669, -2.095) (3.2625, -2.0994) knots 0 0 0 1 1 1
  spline S174 degree 2 poles (3.2625, -2.0994) (3.2579, -2.1038) (3.2579, -2.1096) knots 0 0 0 1 1 1
  spline S175 degree 2 poles (3.2579, -2.1096) (3.2579, -2.1161) (3.2669, -2.1244) (3.2758, -2.1244) knots 0 0 0 1 2 2 2
  spline S176 degree 2 poles (3.2758, -2.1244) (3.2852, -2.1244) (3.301, -2.1154) (3.3077, -2.1025) (3.3077, -2.0921) knots 0 0 0 1 2 3 3 3
  line L123 (3.3077, -2.0921) -> (3.3077, -2.0832)
  line L124 (3.3955, -1.952) -> (3.4523, -1.952)
  line L125 (3.4523, -1.952) -> (3.4523, -2.0549)
  line L126 (3.4523, -2.0549) -> (3.4937, -2.007)
  line L127 (3.4937, -2.007) -> (3.562, -2.007)
  line L128 (3.562, -2.007) -> (3.51, -2.0578)
  line L129 (3.51, -2.0578) -> (3.5651, -2.152)
  line L130 (3.5651, -2.152) -> (3.5025, -2.152)
  line L131 (3.5025, -2.152) -> (3.4731, -2.094)
  line L132 (3.4731, -2.094) -> (3.4523, -2.1142)
  line L133 (3.4523, -2.1142) -> (3.4523, -2.152)
  line L134 (3.4523, -2.152) -> (3.3955, -2.152)
  line L135 (3.3955, -2.152) -> (3.3955, -1.952)
  line L136 (3.6328, -2.0542) -> (3.5797, -2.0486)
  spline S177 degree 2 poles (3.5797, -2.0486) (3.5828, -2.0345) (3.594, -2.0186) (3.6047, -2.0126) knots 0 0 0 1 2 2 2
  spline S178 degree 2 poles (3.6047, -2.0126) (3.6122, -2.0084) (3.639, -2.0037) (3.6546, -2.0037) knots 0 0 0 1 2 2 2
  spline S179 degree 2 poles (3.6546, -2.0037) (3.6794, -2.0037) (3.7096, -2.0093) (3.7198, -2.0182) knots 0 0 0 1 2 2 2
  spline S180 degree 2 poles (3.7198, -2.0182) (3.727, -2.0243) (3.7351, -2.0469) (3.7351, -2.0571) knots 0 0 0 1 2 2 2
  line L137 (3.7351, -2.0571) -> (3.7351, -2.1212)
  spline S181 degree 2 poles (3.7351, -2.1212) (3.7351, -2.1314) (3.7376, -2.1429) (3.742, -2.152) knots 0 0 0 1 2 2 2
  line L138 (3.742, -2.152) -> (3.6898, -2.152)
  spline S182 degree 2 poles (3.6898, -2.152) (3.6867, -2.1464) (3.6848, -2.1406) (3.6838, -2.1342) knots 0 0 0 1 2 2 2
  spline S183 degree 2 poles (3.6838, -2.1342) (3.6731, -2.1446) (3.6623, -2.1493) knots 0 0 0 1 1 1
  spline S184 degree 2 poles (3.6623, -2.1493) (3.6475, -2.1552) (3.628, -2.1552) knots 0 0 0 1 1 1
  spline S185 degree 2 poles (3.628, -2.1552) (3.602, -2.1552) (3.5753, -2.1312) (3.5753, -2.1136) knots 0 0 0 1 2 2 2
  spline S186 degree 2 poles (3.5753, -2.1136) (3.5753, -2.0971) (3.5849, -2.0865) knots 0 0 0 1 1 1
  spline S187 degree 2 poles (3.5849, -2.0865) (3.5947, -2.0759) (3.6207, -2.0707) knots 0 0 0 1 1 1
  spline S188 degree 2 poles (3.6207, -2.0707) (3.6519, -2.0644) (3.6704, -2.0594) (3.6808, -2.0553) knots 0 0 0 1 2 2 2
  spline S189 degree 2 poles (3.6808, -2.0553) (3.6808, -2.0451) (3.6723, -2.0368) (3.6617, -2.0368) knots 0 0 0 1 2 2 2
  spline S190 degree 2 poles (3.6617, -2.0368) (3.6482, -2.0368) (3.6413, -2.0413) knots 0 0 0 1 1 1
  spline S191 degree 2 poles (3.6413, -2.0413) (3.6361, -2.0447) (3.6328, -2.0542) knots 0 0 0 1 1 1
  spline S192 degree 2 poles (3.6808, -2.0832) (3.6694, -2.0873) (3.6569, -2.0905) knots 0 0 0 1 1 1
  spline S193 degree 2 poles (3.6569, -2.0905) (3.64, -2.095) (3.6355, -2.0994) knots 0 0 0 1 1 1
  spline S194 degree 2 poles (3.6355, -2.0994) (3.6309, -2.1038) (3.6309, -2.1096) knots 0 0 0 1 1 1
  spline S195 degree 2 poles (3.6309, -2.1096) (3.6309, -2.1161) (3.64, -2.1244) (3.6488, -2.1244) knots 0 0 0 1 2 2 2
  spline S196 degree 2 poles (3.6488, -2.1244) (3.6582, -2.1244) (3.674, -2.1154) (3.6808, -2.1025) (3.6808, -2.0921) knots 0 0 0 1 2 3 3 3
  line L139 (3.6808, -2.0921) -> (3.6808, -2.0832)
  point P0 (0, 0)
  constraints: 4 other
extrude "Extrusion4" add sketch "Sketch4" along normal blind 0.05 contours L8 S0 S1 S2 S3 L9 S4 S5 S6 S7 S8 S9 | L10 S10 S11 S12 S13 L11 S14 L12 S15 S16 S17 S18 S19 S20 S21 S22 S23 S24 | L14 L15 S30 S31 L16 S32 S33 S34 L17 L18 L19 | L20 L21 L22 L23 | S35 S36 S37 S38 S39 S40 | L24 S45 S46 S47 S48 S49 S50 S51 S52 L25 S53 S54 S55 S56 S57 S58 S59 S60 | L26 S61 S62 S63 L27 L28 | L32 L33 L34 L35 | L36 L37 L38 L39 | L40 S66 S67 S68 S69 L41 S70 L42 S71 S72 S73 S74 S75 S76 S77 S78 S79 S80 | L44 S86 S87 S88 S89 S90 S91 S92 S93 L45 S94 S95 S96 S97 S98 S99 S100 S101 | L46 L47 L48 L49 L50 L51 L52 L53 | L54 L55 L56 L57 L58 L59 L60 L61 L62 L63 L64 L65 | L66 L67 L68 L69 L70 L71 L72 L73 | L77 L78 S102 S103 S104 S105 S106 L79 L80 L81 S107 S108 L82 L83 L84 | L88 S112 S113 S114 S115 L89 S116 S117 S118 S119 S120 S121 | L90 L91 L92 L93
fillet "Face Fillet3" radius 0.133 1 edges at (4, 2.5, 0.1)
fillet "Face Fillet4" radius 0.133 1 edges at (-4, 2.5, 0.1)
fillet "Face Fillet5" radius 0.133 1 edges at (-4, -2.5, 0.1)
fillet "Face Fillet6" radius 0.133 1 edges at (4, -2.5, 0.1)
extrude "Extrusion5" add sketch "Sketch4" along normal blind 0.05 contours L94 S122 S123 S124 S125 S126 S127 S128 S129 L95 S130 S131 S132 S133 S134 S135 S136 S137 | L96 L97 L98 L99 | L100 L101 L102 L103 | L104 L105 L106 L107 L108 L109 L110 | S138 S139 S140 S141 S142 S143 | L111 L112 L113 S148 S149 S150 S151 S152 L114 L115 | L116 L117 L118 L119 | L120 S157 S158 S159 S160 L121 S161 L122 S162 S163 S164 S165 S166 S167 S168 S169 S170 S171 | L124 L125 L126 L127 L128 L129 L130 L131 L132 L133 L134 L135 | L136 S177 S178 S179 S180 L137 S181 L138 S182 S183 S184 S185 S186 S187 S188 S189 S190 S191
body "Solid1"
